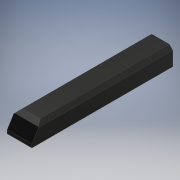
# Autodesk Inventor part: key_black
Saved by Autodesk Inventor 2017 (Build 210142000, 142)
## iProperties
Created: 2018-03-15
Part Number: key_black
Material: Generic
Document SubType Name: Modeling
Designer: Luiz Gustavo
Density: 1 g/cm^3
Appearance: Glossy - Black
Author: Luiz Gustavo
Autodesk Inventor part; units mm, degrees
ref_plane "YZ Plane" through (0, 0, 0) normal (1, 0, 0) x (0, 1, 0)
ref_plane "XZ Plane" through (0, 0, 0) normal (0, 1, 0) x (-1, 0, 0)
ref_plane "XY Plane" through (0, 0, 0) normal (0, 0, 1) x (1, 0, 0)
sketch "Sketch1" plane through (0, 0, 0) normal (0, 0, 1) x (1, 0, 0)
  line L0 (-7, -40) -> (7, -40)
  line L1 (7, -40) -> (7, 40)
  line L2 (7, 40) -> (-7, 40)
  line L3 (-7, 40) -> (-7, -40)
  line L4 (-7, -40) -> (7, 40) construction
  line L5 (7, -40) -> (-7, 40) construction
  point P0 (0, 0)
  dimension "d0" = 14
  dimension "d1" = 80
  constraints: 12 end point, 2 midpoint, 2 parallel, 1 horizontal, 1 perpendicular
  measures "d0" distance of L1.end L2.end
  measures "d1" distance between parallel lines of L0 L2
extrude "Extrusion1" add sketch "Sketch1" along normal blind 10
chamfer "Chamfer1" distance 5 distance2 8 1 edges at (0, -40, 10) measured on face at (-2.3333, 13.3333, 10)
chamfer "Chamfer2" distance 2 angle 45 3 edges at (7, 2.5, 10) (-7, 2.5, 10) (0, -35, 10)
equation "\"d0\" = 2 * blackkey_halfwidth"
equation "\"d1\" = blackkey_length"
equation "\"d2\" = 0.5 * key_height"
equation "\"blackkey_halfwidth\" = 7"
equation "\"blackkey_length\" = 80"
equation "\"key_height\" = 20"
body "Solid1"
